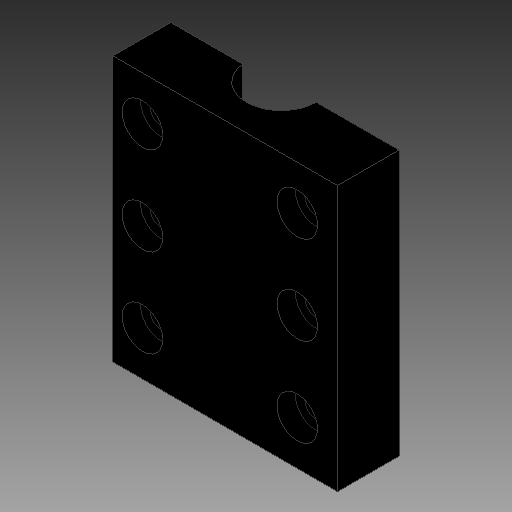
# Autodesk Inventor part: J007580
Saved by Autodesk Inventor 2018.2 (Build 222227000, 227)
## iProperties
Created: 2018-07-18
Part Number: J007580
Material: ALUMINUM, 6061-T651
Document SubType Name: Modeling
Designer: legant_local
Density: 2.7 g/cm^3
Appearance: Anodized - Black
Description: xgalvo_to_base_clamp
Project: P-303502
Vendor: HHMI: JRC - JET
Catalog Web Link: MPFI custom
Stock Number: J007580
ALTERED ITEM PART NUMBER: N/A
ALTERED ITEM VENDOR: N/A
ALTERED ITEM DESCRIPTION: N/A
DESIGN DEPARTMENT: HHMI: JRC - ID&F
LAB/DEPT: BETZIG (LAB)
REQUESTING SCIENTIST: BETZIG, ERIC
SPECIAL FINISH: ANODIZE PER MIL-A-8625F, TYPE II, CLASS 2 (BLACK)
SURFACE ROUGHNESS: 32 Ra
Author: legant_local
Revision Number: 0
Autodesk Inventor part; units mm, degrees
ref_plane "YZ Plane" through (0, 0, 0) normal (1, 0, 0) x (0, 1, 0)
ref_plane "XZ Plane" through (0, 0, 0) normal (0, 1, 0) x (-1, 0, 0)
ref_plane "XY Plane" through (0, 0, 0) normal (0, 0, 1) x (1, 0, 0)
sketch "Sketch1" plane through (0, 0, 0) normal (0, 0, 1) x (1, 0, 0)
  line L0 (-15.25, 18) -> (15.25, 18)
  line L1 (15.25, 18) -> (15.25, -18)
  line L2 (15.25, -18) -> (-15.25, -18)
  line L3 (-15.25, -18) -> (-15.25, 18)
  point P0 (0, 0)
  dimension "d0" = 30.5
  dimension "d1" = 36
  dimension "d2" = 18
  dimension "d3" = 15.25
  constraints: 8 end point, 2 parallel, 1 horizontal, 1 perpendicular
  measures "d0" distance of L1.end L2.end
  measures "d1" distance of L0.end L1.end
  measures "d2" distance from line of L0 point (0, 0)
  measures "d3" distance from line of L3 point (0, 0)
extrude "Extrusion1" add sketch "Sketch1" along normal blind 8.35
sketch "Sketch2" plane through (-15.25, 18, 0) normal (0, 1, 0) x (1, 0, 0)
  line L0 (30.5, 0) -> (30.5, -8.35) projected
  line L1 (30.5, -8.35) -> (70.5, -8.35) projected
  line L2 (70.5, 11.65) -> (70.5, -8.35) projected
  line L3 (0, 11.65) -> (70.5, 11.65) projected
  line L4 (0, 11.65) -> (0, 0.5) projected
  line L5 (0, 0.5) -> (9.7766, 0.5) projected
  arc A0 (19.2498, 0) -> (9.7766, 0.5) centre (14.5, 0) ccw projected
  line L6 (19.2498, 0) -> (30.5, 0) projected
  circle A1 centre (40.5, 1.65) radius 0.847 projected
  circle A2 centre (62.5, 1.65) radius 0.847 projected
  circle A3 centre (54.5, 1.65) radius 4 projected
  circle A4 centre (14.5, 0) radius 4.7498
  point P0 (15.25, 0)
  constraints: 1 coincident, 1 horizontal alignment, 2 other
extrude "Extrusion2" cut sketch "Sketch2" against normal through all contours A4 A0
sketch "Sketch3" plane through (0, 0, 8.35) normal (0, 0, 1) x (1, 0, 0)
  circle A0 centre (-11.25, 12) radius 1.0065 projected
  circle A1 centre (-11.25, 0) radius 1.0065 projected
  circle A2 centre (-11.25, -12) radius 1.0065 projected
  circle A3 centre (9.7764, 12) radius 1.0065 projected
  circle A4 centre (9.7764, 0) radius 1.0065 projected
  circle A5 centre (9.7764, -12) radius 1.0065 projected
  point P0 (0, 0)
hole "CBore for M2.5 screw" at (-11.25, -12, 8.35) at (-11.25, 0, 8.35) at (-11.25, 12, 8.35) at (9.7764, -12, 8.35) at (9.7764, 0, 8.35) at (9.7764, 12, 8.35) direction (0, 0, -1) diameter 2.9 end through all counterbore diameter 5.5 counterbore depth 2.5 clearance for "Socket Head Cap Screw" size "M2.5" standard "Ansi Metric M Profile"
sketch "Sketch4" plane through (0, 0, 0) normal (0, 0, -1) x (-1, 0, 0)
  circle A0 centre (11.25, 0) radius 1.45 projected
  circle A1 centre (11.25, -12) radius 1.45 projected
  circle A2 centre (11.25, 12) radius 1.45 projected
  line L0 (5.4998, 18) -> (5.4998, -18) projected
  line L1 (5.4998, -18) -> (15.25, -18) projected
  line L2 (15.25, -18) -> (15.25, 18) projected
  line L3 (15.25, 18) -> (5.4998, 18) projected
  line L4 (15.25, -18) -> (4.4998, -18)
  line L5 (4.4998, -18) -> (4.4998, 18)
  line L6 (4.4998, 18) -> (15.25, 18)
  line L7 (15.25, 18) -> (15.25, -18)
  point P0 (0, 0)
  dimension "d17" = 1
  constraints: 8 end point, 2 parallel, 1 horizontal, 1 perpendicular
  measures "d17" distance between parallel lines of L0 L5
extrude "Extrusion3" cut sketch "Sketch4" against normal blind 0.5
equation "\"d2\" = 0.5 * d1"
equation "\"d3\" = 0.5 * d0"
body "Solid1"
